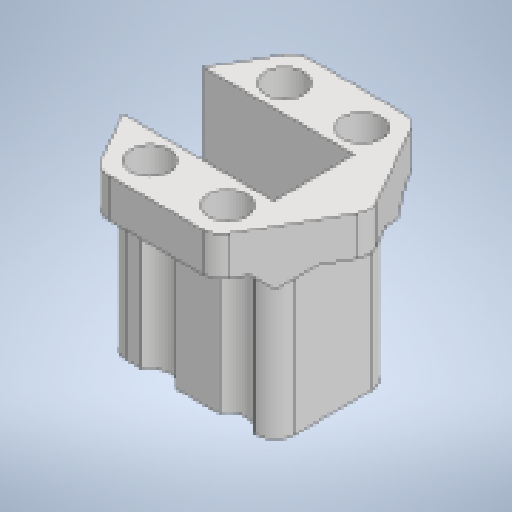
# Autodesk Inventor part: Switch Holder
Saved by Autodesk Inventor 2023.2 (Build 272271000, 271)
## iProperties
Created: 2023-03-17
Part Number: Switch Holder
Material: Generic
Document SubType Name: Modeling
Designer: Nathan Cai
Density: 1 g/cm^3
Appearance: Default
Author: Nathan Cai
Autodesk Inventor part; units mm, degrees
ref_plane "YZ Plane" through (0, 0, 0) normal (1, 0, 0) x (0, 1, 0)
ref_plane "XZ Plane" through (0, 0, 0) normal (0, 1, 0) x (-1, 0, 0)
ref_plane "XY Plane" through (0, 0, 0) normal (0, 0, 1) x (1, 0, 0)
sketch "Sketch1" plane through (0, 0, 0) normal (0, 1, 0) x (-1, 0, 0)
  circle A0 centre (0, 0) radius 6.35 construction
  line L0 (0, 0) -> (6.35, 0) construction
  circle A1 centre (6.35, 0) radius 1.5875
  circle A2 centre (3.175, 5.4993) radius 1.5875
  circle A3 centre (-3.175, 5.4993) radius 1.5875
  circle A4 centre (-6.35, 0) radius 1.5875
  circle A5 centre (-3.175, -5.4993) radius 1.5875
  circle A6 centre (3.175, -5.4993) radius 1.5875
  line L1 (9.525, 0) -> (4.7625, -8.2489)
  line L2 (4.7625, -8.2489) -> (-4.7625, -8.2489)
  line L3 (-4.7625, -8.2489) -> (-9.525, 0)
  line L4 (-9.525, 0) -> (-4.7625, 8.2489)
  line L5 (-4.7625, 8.2489) -> (4.7625, 8.2489)
  line L6 (4.7625, 8.2489) -> (9.525, 0)
  dimension "d0" = 12.7
  dimension "d1" = 3.175
  dimension "d4" = 360
  dimension "d6" = 9.525
  constraints: 14 end point, 6 centre point, 3 coincident, 1 horizontal, 1 horizontal alignment, 1 point on line, 28 other
  measures "d1" diameter of A1
  measures "d6" distance of point (0, 0) L1.start
extrude "Extrusion1" add sketch "Sketch1" along normal blind 15.875 contours A1 | A4 | L1 L2 L3 L4 L5 L6
sketch "Sketch2" plane through (0, 15.875, 0) normal (0, 1, 0) x (1, 0, 0)
  line L0 (-9.525, 0) -> (-4.7625, -8.2489) projected
  line L1 (-9.525, 0) -> (0, 0) construction
  line L2 (-7.9375, -3.302) -> (4.7625, -3.302)
  line L3 (4.7625, -3.302) -> (4.7625, 3.302)
  line L4 (4.7625, 3.302) -> (-7.9375, 3.302)
  line L5 (-7.9375, 3.302) -> (-7.9375, -3.302) construction
  line L6 (-7.9375, -3.302) -> (4.7625, 3.302) construction
  line L7 (4.7625, -3.302) -> (-7.9375, 3.302) construction
  line L8 (-4.7625, -8.2489) -> (4.7625, -8.2489) projected
  line L9 (4.7625, -8.2489) -> (9.525, 0) projected
  line L10 (9.525, 0) -> (4.7625, 8.2489) projected
  line L11 (4.7625, 8.2489) -> (-4.7625, 8.2489) projected
  line L12 (-4.7625, 8.2489) -> (-9.525, 0) projected
  line L13 (-9.525, 0) -> (-4.7625, -8.2489) projected
  circle A0 centre (-3.175, -5.4993) radius 1.5875 projected
  circle A1 centre (3.175, -5.4993) radius 1.5875 projected
  circle A2 centre (3.175, 5.4993) radius 1.5875 projected
  circle A3 centre (-3.175, 5.4993) radius 1.5875 projected
  point P0 (-1.5875, 0)
  point P1 (-7.6186, 3.302)
  point P2 (-7.6186, -3.302)
  dimension "d9" = 12.7
  dimension "d10" = 6.604
  dimension "d11" = 4.7625
  constraints: 14 end point, 2 horizontal, 2 midpoint, 2 parallel, 1 perpendicular, 1 point on line
  measures "d9" distance of L4.end L3.end
  measures "d10" distance of L3.end L2.end
  measures "d11" distance from line of L9.end L3
extrude "Extrusion2" cut sketch "Sketch2" against normal blind 12.7 contours L12 L4 L3 L2 L0
sketch "Sketch3" plane through (0, 0, 0) normal (0, -1, 0) x (1, 0, 0)
  line L0 (6.35, 4.7625) -> (-9.525, 4.7625)
  line L1 (-9.525, 4.7625) -> (-9.525, -4.7625)
  line L2 (-9.525, -4.7625) -> (6.35, -4.7625)
  line L3 (6.35, -4.7625) -> (6.35, 4.7625)
  line L4 (6.35, 4.7625) -> (-9.525, -4.7625) construction
  line L5 (-9.525, 4.7625) -> (6.35, -4.7625) construction
  line L6 (-4.7625, 8.2489) -> (4.7625, 8.2489) projected
  line L7 (-9.525, 0) -> (-4.7625, 8.2489) projected
  line L8 (-4.7625, -8.2489) -> (-9.525, 0) projected
  line L9 (4.7625, -8.2489) -> (-4.7625, -8.2489) projected
  line L10 (9.525, 0) -> (4.7625, -8.2489) projected
  line L11 (4.7625, 8.2489) -> (9.525, 0) projected
  circle A0 centre (-3.175, 5.4993) radius 1.5875 projected
  circle A1 centre (3.175, 5.4993) radius 1.5875 projected
  circle A2 centre (3.175, -5.4993) radius 1.5875 projected
  circle A3 centre (-3.175, -5.4993) radius 1.5875 projected
  line L12 (6.35, 0) -> (-9.525, 0) construction
  point P0 (0, 0)
  point P1 (-1.5875, 0)
  point P2 (4.5812, -4.7625)
  point P3 (1.7688, -4.7625)
  point P4 (-1.7688, -4.7625)
  point P5 (-4.5812, -4.7625)
  point P6 (-6.7754, -4.7625)
  point P7 (-6.7754, 4.7625)
  point P8 (-4.5812, 4.7625)
  point P9 (-1.7688, 4.7625)
  point P10 (1.7688, 4.7625)
  point P11 (4.5812, 4.7625)
  dimension "d14" = 15.875
  dimension "d15" = 9.525
  dimension "d16" = 3.175
  constraints: 14 end point, 3 midpoint, 2 horizontal, 2 parallel, 1 perpendicular
  measures "d14" distance of L2.end L1.end
  measures "d15" distance of L1.end L0.end
  measures "d16" distance from line of L10.start L3
extrude "Extrusion3" cut sketch "Sketch3" against normal blind 12.7 contours L0 A1 A0 L7 L6 L11 L10 L9 L8 L2 A3 A2 L3
chamfer "Chamfer1" distance 1.5875 angle 45 7 edges at (-5.6783, 12.7, 4.7625) (0, 12.7, 4.7625) (5.4656, 12.7, 4.7625) (6.35, 12.7, 0) (5.4656, 12.7, -4.7625) (0, 12.7, -4.7625) (-5.6783, 12.7, -4.7625)
fillet "Fillet1" radius 1.5875 10 edges at (-4.7625, 14.2875, 8.2489) (4.7625, 14.2875, 8.2489) (9.525, 14.2875, 0) (4.7625, 14.2875, -8.2489) (-4.7625, 14.2875, -8.2489) (6.35, 5.5562, 4.7625) (6.35, 5.5562, -4.7625) (-6.7754, 5.5562, 4.7625) (-6.7754, 5.5562, -4.7625) (-9.525, 1.5875, 0)
body "Solid1"
